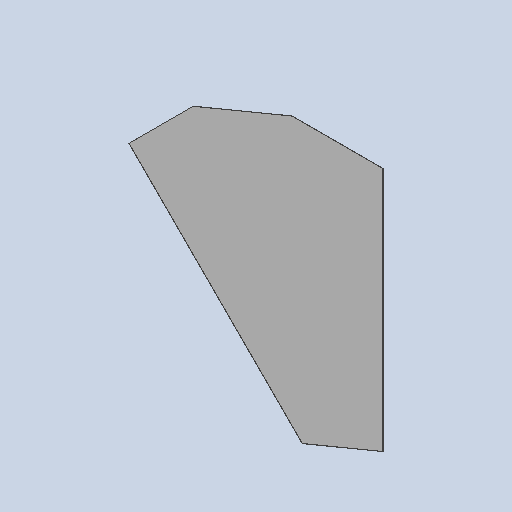
# Autodesk Inventor part: DMF 01 57 Сетка кассеты v2.1
Saved by Autodesk Inventor 2025 (Build 290162010, 162A)
## iProperties
Created: 2024-05-05
Part Number: DMF 01 57 Сетка кассеты v2.1
Material: Generic
Document SubType Name: Sheet Metal
Designer: pokla
Density: 1 g/cm^3
Appearance: Default
Sheet Metal Rule: Default
Author: pokla
Autodesk Inventor part; units mm, degrees
ref_plane "YZ Plane" through (0, 0, 0) normal (1, 0, 0) x (0, 1, 0)
ref_plane "XZ Plane" through (0, 0, 0) normal (0, 1, 0) x (-1, 0, 0)
ref_plane "XY Plane" through (0, 0, 0) normal (0, 0, 1) x (1, 0, 0)
sketch "Sketch1" plane through (0, 0, 0) normal (0, 0, 1) x (1, 0, 0)
  line L0 (0, 277.6336) -> (196.3166, 196.3166) construction
  line L1 (196.3166, 196.3166) -> (277.6336, 0) construction
  line L2 (277.6336, 0) -> (196.3166, -196.3166) construction
  line L3 (196.3166, -196.3166) -> (0, -277.6336) construction
  line L4 (0, -277.6336) -> (-196.3166, -196.3166) construction
  line L5 (-196.3166, -196.3166) -> (-277.6336, 0) construction
  line L6 (-277.6336, 0) -> (-196.3166, 196.3166) construction
  line L7 (-196.3166, 196.3166) -> (0, 277.6336)
  line L8 (-196.3166, 196.3166) -> (0, 277.6336)
  line L9 (-461.2666, 773.8898) -> (-221.0579, 873.3874)
  line L10 (-98.1583, 236.9751) -> (-341.1623, 823.6386) construction
  line L11 (-221.0579, 873.3874) -> (0, 873.3874)
  line L12 (0, 873.3874) -> (0, 277.6336)
  line L13 (-461.2666, 773.8898) -> (-617.5782, 617.5782)
  line L14 (-617.5782, 617.5782) -> (-196.3166, 196.3166)
  point P0 (0, 0)
  point P1 (0, 0)
  dimension "d0" = 513
  dimension "d2" = 260
  dimension "d3" = 635
  constraints: 30 end point, 2 midpoint, 1 coincident, 1 horizontal, 1 parallel, 1 perpendicular, 1 symmetric about line, 1 vertical, 1 vertical alignment, 17 other
  measures "d0" distance between parallel lines of L5 L1
  measures "d2" distance of L9.start L9.end
  measures "d3" distance of L10.end L10.start
extrude "Extrusion1" add sketch "Sketch1" along normal mid plane 0.5
sketch "Sketch7" plane through (0, 0, 0.25) normal (0, 0, 1) x (1, 0, 0)
  line L0 (-13, 868.3874) -> (-5, 868.3874)
  line L1 (-5, 868.3874) -> (-5, 860.3874)
  line L2 (-5, 860.3874) -> (-13, 860.3874)
  line L3 (-13, 860.3874) -> (-13, 868.3874)
  line L4 (0, 873.3874) -> (-221.0579, 873.3874) projected
  line L5 (0, 277.6336) -> (0, 873.3874) projected
  point P0 (0, 0)
  dimension "d54" = 8
  dimension "d55" = 8
  dimension "d56" = 5
  dimension "d57" = 5
  constraints: 8 end point, 2 parallel, 1 horizontal, 1 perpendicular
  measures "d54" distance of L1.end L2.end
  measures "d55" distance of L0.end L1.end
  measures "d56" distance between parallel lines of L4 L0
  measures "d57" distance between parallel lines of L5 L1
extrude "Extrusion5" [suppressed]
pattern_linear "Rectangular Pattern1" [suppressed]
equation "\"d0\" = Барабан_габарит_по_кассетам"
equation "\"d2\" = Кассета_длина_грани"
equation "\"d3\" = Кассета_высота"
equation "\"BendRadius\" = Thickness"
equation "\"BendReliefWidth\" = Thickness"
equation "\"BendReliefDepth\" = 0.5 * Thickness"
equation "\"CornerReliefSize\" = 4 * Thickness"
equation "\"MinimumRemnant\" = 2 * Thickness"
equation "\"TransitionRadius\" = BendRadius"
equation "\"JacobiRadiusSize\" = BendRadius"
equation "\"GapSize\" = Thickness"
equation "\"Барабан_габарит_по_кассетам\" = 513"
equation "\"Кассета_длина_грани\" = 260"
equation "\"Кассета_высота\" = 635"
equation "\"Thickness\" = 0.5"
body "Solid1"
